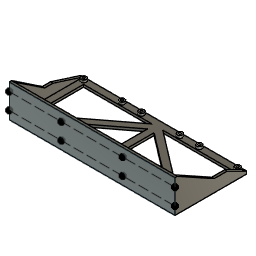
motor-driver-mount (Autodesk Fusion 360 design; units mm, degrees)
Autodesk Fusion 360 part; units mm, degrees
note: some values were not read from the file. Set by a fixed rule: which sketch regions a step uses.
sketch "Sketch1" plane through (0, 0, 0) normal (0, 0, 1) x (1, 0, 0)
  line L0 (0, 0) -> (203, 0)
  line L1 (203, 0) -> (203, 88)
  line L2 (203, 88) -> (0, 88)
  line L3 (0, 88) -> (0, 0)
  line L4 (3, 3) -> (200, 3)
  line L5 (200, 3) -> (200, 88)
  line L6 (200, 88) -> (3, 88)
  line L7 (3, 88) -> (3, 3)
  line L8 (3, 45.5) -> (200, 45.5) construction
  line L9 (101.5, 88) -> (101.5, 3) construction
  line L10 (3, 84) -> (101.5, 84) construction
  circle A0 centre (7.25, 84) radius 1.75 construction
  circle A1 centre (7.25, 84) radius 1.4
  circle A2 centre (54.25, 84) radius 1.4
  circle A3 centre (78, 84) radius 1.4
  line L11 (101.5, 80) -> (3, 80)
  line L12 (11, 88) -> (11, 45.5)
  line L13 (101.5, 80) -> (200, 80)
  line L14 (192, 88) -> (192, 45.5)
  circle A4 centre (195.75, 84) radius 1.4
  circle A5 centre (148.75, 84) radius 1.4
  circle A6 centre (125, 84) radius 1.4
  line L15 (11, 3) -> (11, 45.5)
  line L16 (101.5, 11) -> (3, 11)
  circle A7 centre (7.25, 7) radius 1.4
  circle A8 centre (54.25, 7) radius 1.4
  circle A9 centre (78, 7) radius 1.4
  circle A10 centre (125, 7) radius 1.4
  circle A11 centre (148.75, 7) radius 1.4
  line L17 (101.5, 11) -> (200, 11)
  line L18 (192, 3) -> (192, 45.5)
  circle A12 centre (195.75, 7) radius 1.4
  line L19 (11, 16.03) -> (94.9027, 80)
  line L20 (17.5973, 11) -> (101.5, 74.97)
  line L21 (101.5, 80) -> (11, 11) construction
  line L22 (97.5, 80) -> (97.5, 11)
  line L23 (105.5, 80) -> (105.5, 11)
  line L24 (185.4027, 11) -> (101.5, 74.97)
  line L25 (192, 16.03) -> (108.0973, 80)
  circle A13 centre (7.25, 84) radius 3.25
  circle A14 centre (54.25, 84) radius 3.25
  circle A15 centre (78, 84) radius 3.25
  circle A16 centre (195.75, 84) radius 3.25
  circle A17 centre (148.75, 84) radius 3.25
  circle A18 centre (125, 84) radius 3.25
  circle A19 centre (7.25, 7) radius 3.25
  circle A20 centre (54.25, 7) radius 3.25
  circle A21 centre (78, 7) radius 3.25
  circle A22 centre (125, 7) radius 3.25
  circle A23 centre (148.75, 7) radius 3.25
  circle A24 centre (195.75, 7) radius 3.25
  dimension "d1" = 3
  dimension "d2" = 3
  dimension "d3" = 3
  dimension "d4" = 197
  dimension "d5" = 85
  dimension "d6" = 4
  dimension "d7" = 3.5
  dimension "d8" = 2.5
  dimension "d10" = 2.8
  dimension "d11" = 47
  dimension "d13" = 23.5
  dimension "d14" = 8
  dimension "d15" = 8
  dimension "d16" = 8
  dimension "d17" = 4
  dimension "d18" = 4
  dimension "d21" = 6.5
  constraint horizontal L0
  constraint vertical L1
  constraint horizontal L2
  constraint vertical L3
  constraint coincident L0.start L3.end
  constraint horizontal L4
  constraint vertical L5
  constraint horizontal L6
  constraint vertical L7
  constraint coincident L2 L5.end
  constraint midpoint L7 L8.start
  constraint midpoint L5 L8.end
  constraint midpoint L2 L9.start
  constraint midpoint L4 L9.end
  constraint coincident L7 L10.start
  constraint coincident L9 L10.end
  constraint perpendicular L9 L10
  constraint coincident L10 A0.centre
  constraint concentric A0 A1
  constraint coincident L10 A2.centre
  constraint coincident L10 A3.centre
  constraint equal A2 A3
  constraint equal A1 A3
  constraint coincident L9 L11.start
  constraint coincident L7 L11.end
  constraint perpendicular L7 L11
  constraint coincident L6 L12.start
  constraint coincident L8 L12.end
  constraint perpendicular L8 L12
  constraint symmetric L9 A1 A4
  constraint symmetric L9 A2 A5
  constraint symmetric L9 A3 A6
  constraint symmetric L9 L11.start L13.start
  constraint symmetric L9 L11.end L13.end
  constraint symmetric L9 L12.start L14.start
  constraint symmetric L9 L12.end L14.end
  constraint symmetric L8 A1 A7
  constraint symmetric L8 A2 A8
  constraint symmetric L8 A3 A9
  constraint symmetric L8 L11.start L16.start
  constraint symmetric L8 L11.end L16.end
  constraint symmetric L8 L12.start L15.start
  constraint symmetric L8 L12.end L15.end
  constraint symmetric L8 L13.end L17.end
  constraint symmetric L8 L14.start L18.start
  constraint symmetric L8 L14.end L18.end
  constraint symmetric L8 A4 A12
  constraint symmetric L8 A5 A11
  constraint symmetric L8 A6 A10
  constraint coincident L15 L19.start
  constraint coincident L11 L19.end
  constraint coincident L16 L20.start
  constraint coincident L9 L20.end
  constraint parallel L19 L20
  constraint coincident L15 L21.end
  constraint coincident L16 L21.end
  constraint parallel L20 L21
  constraint coincident L11 L22.start
  constraint coincident L16 L22.end
  constraint perpendicular L16 L22
  constraint symmetric L9 L19.start L25.start
  constraint symmetric L9 L19.end L25.end
  constraint symmetric L9 L20.start L24.start
  constraint symmetric L9 L20.end L24.end
  constraint symmetric L9 L22.start L23.start
  constraint symmetric L9 L22.end L23.end
  constraint concentric A1 A13
  constraint concentric A2 A14
  constraint concentric A3 A15
  constraint equal A13 A14
  constraint equal A14 A15
  constraint symmetric L9 A13 A16
  constraint symmetric L9 A14 A17
  constraint symmetric L9 A15 A18
  constraint symmetric L8 A13 A19
  constraint symmetric L8 A14 A20
  constraint symmetric L8 A15 A21
  constraint symmetric L8 A16 A24
  constraint symmetric L8 A17 A23
  constraint symmetric L8 A18 A22
  measures "d1" distance of L0 L4
  measures "d2" distance of L3 L7
  measures "d3" distance of L1 L5
  measures "d4" distance of L5 L7
  measures "d5" distance of L4 L6
  measures "d6" distance of L2 L10
  measures "d7" diameter of A0
  measures "d8" distance of L7 A0
  measures "d10" diameter of A1
  measures "d11" distance of A0.centre A2.centre
  measures "d13" distance of L9 A3.centre
  measures "d14" distance of L2 L11
  measures "d15" distance of L7 L12
  measures "d16" distance of L19 L20
  measures "d17" distance of L19 L21
  measures "d18" distance of L9 L22
  measures "d21" diameter of A13
extrude "Extrude1" add sketch "Sketch1" along normal blind 3 contours L2 L6 L7 L11 L12 | L2 L5 L6 L13 L14 | L2 L6 L11 L12 L13 L14 | L7 L11 L12 L15 L16 | L5 L13 L14 L17 L18 | L4 L7 L15 L16 | L4 L5 L17 L18 | L11 L15 L16 L19 L20 L22 | L4 L15 L16 L17 L18 | L13 L17 L18 L23 L24 L25 | L11 L13 L20 L22 L23 L24 | L16 L17 L20 L22 L23 L24 | A13 | A14 | A15 | A16 | A17 | A18 | A19 | A20 | A21 | A22 | A23 | A24
extrude "Extrude2" add sketch "Sketch1" along normal blind 6 contours A13 | A14 | A15 | A16 | A17 | A18 | A19 | A20 | A21 | A22 | A23 | A24
extrude "Extrude3" add sketch "Sketch1" along normal blind 40 contours L0 L1 L2 L3 L4 L5 L7
sketch "Sketch2" plane through (3, 0, 0) normal (1, 0, 0) x (0, 1, 0)
  line L0 (3, 40) -> (3, 3)
  line L1 (3, 3) -> (88, 3)
  line L2 (88, 3) -> (88, 40)
  line L3 (88, 40) -> (3, 40)
  line L4 (45.5, 15) -> (50.5, 15)
  line L5 (3, 40) -> (40.5, 15)
  line L6 (50.5, 15) -> (88, 3)
  line L7 (45.5, 3) -> (45.5, 15) construction
  line L8 (40.5, 15) -> (45.5, 15)
  dimension "d28" = 12
  dimension "d29" = 5
  dimension "d30" = 5
  constraint coincident L0.start L3.end
  constraint coincident L1.end L2.start
  constraint midpoint L1 L7.start
  constraint perpendicular L4 L7
  constraint perpendicular L7 L8
  measures "d28" distance of L1 L4
  measures "d29" distance of L5.end L4.start
  measures "d30" distance of L4.end L4.start
extrude "Extrude4" cut sketch "Sketch2" against normal up to surface (3 mm away) contours L2 L3 L4 L5 L6 L8
sketch "Sketch3" plane through (200, 0, 0) normal (-1, 0, 0) x (0, -1, 0)
  line L0 (-88, 3) -> (-3, 3)
  line L1 (-3, 3) -> (-3, 40)
  line L2 (-3, 40) -> (-88, 40)
  line L3 (-88, 40) -> (-88, 3)
  line L4 (-88, 3) -> (-64, 15)
  line L5 (-64, 15) -> (-48, 15)
  line L6 (-48, 15) -> (-3, 40)
  line L7 (-48, 15) -> (-3, 15) construction
  dimension "d33" = 12
  dimension "d34" = 45
  dimension "d35" = 16
  constraint coincident L0.start L3.end
  constraint perpendicular L3 L5
  constraint coincident L1.end L2.start
  constraint coincident L1 L7.end
  constraint perpendicular L1 L7
  measures "d33" distance of L0 L5
  measures "d34" distance of L5.end L7.end
  measures "d35" distance of L4.end L5.end
extrude "Extrude5" cut sketch "Sketch3" against normal up to surface (3 mm away) contours L2 L3 L4 L5 L6
sketch "Sketch4" plane through (0, 0, 0) normal (0, -1, 0) x (1, 0, 0)
  line L0 (0, 0) -> (203, 0)
  line L1 (203, 0) -> (203, 40)
  line L2 (203, 40) -> (0, 40)
  line L3 (0, 40) -> (0, 0)
  line L4 (0, 30) -> (203, 30) construction
  line L5 (0, 10) -> (203, 10) construction
  circle A0 centre (64, 30) radius 2.5
  circle A1 centre (139, 30) radius 2.5
  circle A2 centre (64, 10) radius 2.5
  circle A3 centre (139, 10) radius 2.5
  dimension "d38" = 10
  dimension "d39" = 20
  dimension "d40" = 5
  dimension "d41" = 64
  dimension "d42" = 64
  dimension "d43" = 64
  dimension "d44" = 64
  constraint coincident L3 L4.start
  constraint coincident L1 L4.end
  constraint perpendicular L1 L4
  constraint coincident L3 L5.start
  constraint coincident L1 L5.end
  constraint perpendicular L1 L5
  constraint coincident L4 A0.centre
  constraint coincident L4 A1.centre
  constraint coincident L5 A2.centre
  constraint coincident L5 A3.centre
  constraint equal A2 A3
  constraint equal A1 A3
  constraint equal A0 A1
  measures "d38" distance of L2 L4
  measures "d39" distance of L4 L5
  measures "d40" diameter of A0
  measures "d41" distance of L3 A0.centre
  measures "d42" distance of L3 A2.centre
  measures "d43" distance of L1 A1.centre
  measures "d44" distance of L1 A3.centre
extrude "Extrude6" cut sketch "Sketch4" against normal up to surface (3 mm away) contours A0 | A1 | A2 | A3
equation "d13 = ( 47 / 2 ) * 1 mm"
